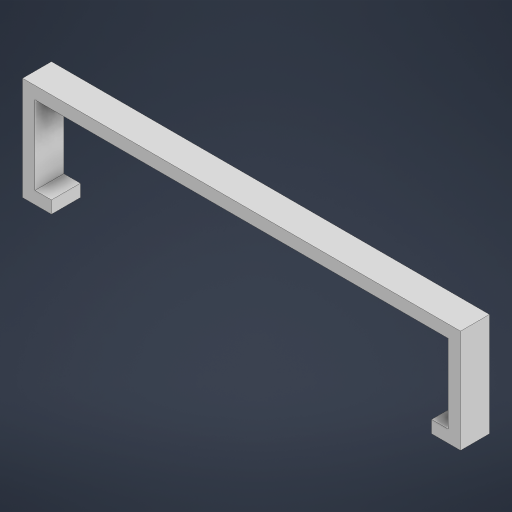
# Autodesk Inventor part: uchwyt
Saved by Autodesk Inventor 2023 (Build 270158000, 158)
## iProperties
Created: 2023-11-16
Part Number: uchwyt
Material: Ogólny
Document SubType Name: Modeling
Designer: mt150
Density: 1 g/cm^3
Appearance: Domyślna
Author: mt150
Autodesk Inventor part; units mm, degrees
ref_plane "YZ Plane" through (0, 0, 0) normal (1, 0, 0) x (0, 1, 0)
ref_plane "XZ Plane" through (0, 0, 0) normal (0, 1, 0) x (-1, 0, 0)
ref_plane "XY Plane" through (0, 0, 0) normal (0, 0, 1) x (1, 0, 0)
sketch "Szkic1" plane through (0, 0, 0) normal (0, 1, 0) x (-1, 0, 0)
  point P0 (0, 0)
sketch "Szkic2" plane through (0, 0, 0) normal (0, 1, 0) x (-1, 0, 0)
  line L0 (0, 0) -> (-100, 0)
  line L1 (-100, 0) -> (-100, 7)
  line L2 (-100, 7) -> (0, 7)
  line L3 (0, 7) -> (0, 0)
  dimension "d0" = 100
  dimension "d1" = 7
  constraints: 8 end point, 2 parallel, 1 horizontal, 1 perpendicular
  measures "d0" distance of L1.end L2.end
  measures "d1" distance of L0.end L1.end
extrude "Wyciągnięcie proste1" add sketch "Szkic2" along normal blind 3
sketch "Szkic3" plane through (0, 3, 0) normal (0, 1, 0) x (1, 0, 0)
  line L0 (0, 0) -> (-3, 0)
  line L1 (-3, 0) -> (-3, -7)
  line L2 (-3, -7) -> (0, -7)
  line L3 (0, -7) -> (0, 0)
  line L4 (100, -7) -> (100, 0) projected
  line L5 (100, 0) -> (103, 0)
  line L6 (103, 0) -> (103, -7)
  line L7 (103, -7) -> (100, -7)
  line L8 (100, -7) -> (100, 0)
  dimension "d4" = 3
  dimension "d5" = 7
  dimension "d6" = 3
  constraints: 16 end point, 4 parallel, 2 horizontal, 2 perpendicular
  measures "d4" distance of L2.end L1.end
  measures "d5" distance of L0.end L1.end
  measures "d6" distance of L6.end L7.end
extrude "Wyciągnięcie proste2" add sketch "Szkic3" against normal blind 22
sketch "Szkic4" plane through (0, -19, 0) normal (0, -1, 0) x (1, 0, 0)
  line L0 (-3, 0) -> (0, 0) projected
  line L1 (-3, 0) -> (4, 0)
  line L2 (4, 0) -> (4, 7)
  line L3 (4, 7) -> (-3, 7)
  line L4 (-3, 7) -> (-3, 0)
  line L5 (100, 0) -> (103, 0) projected
  line L6 (103, 0) -> (96, 0)
  line L7 (96, 0) -> (96, 7)
  line L8 (96, 7) -> (103, 7)
  line L9 (103, 7) -> (103, 0)
  dimension "d9" = 7
  dimension "d10" = 7
  constraints: 16 end point, 4 parallel, 2 horizontal, 2 perpendicular, 1 point on line
  measures "d9" distance of L3.end L2.end
  measures "d10" distance of L7.end L8.end
extrude "Wyciągnięcie proste3" add sketch "Szkic4" along normal blind 3
